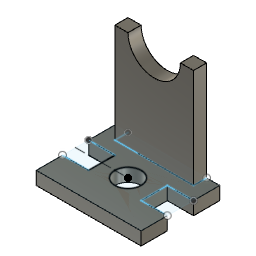
Model 5 (Autodesk Fusion 360 design; units mm, degrees)
Autodesk Fusion 360 part; units mm, degrees
sketch "Sketch15" plane through (0, 0, 0) normal (0, 0, 1) x (1, 0, 0)
  line L0 (0, 0) -> (200, 0)
  line L1 (200, 0) -> (200, 150)
  line L2 (200, 150) -> (0, 150)
  line L3 (0, 150) -> (0, 0)
  dimension "d98" = 200
  dimension "d99" = 150
  constraint horizontal L0
  constraint vertical L1
  constraint horizontal L2
  constraint vertical L3
  constraint coincident L0.start L3.end
  measures "d98" distance of L0.start L0.end
  measures "d99" distance of L0.start L2.end
extrude "Extrude13" add sketch "Sketch15" along normal blind 25
sketch "Sketch16" plane through (0, 0, 25) normal (0, 0, 1) x (-1, 0, 0)
  line L0 (0, -150) -> (0, 0)
  line L1 (0, 0) -> (-200, 0)
  line L2 (-200, 0) -> (-200, -150)
  line L3 (-200, -150) -> (0, -150)
  line L4 (-200, -50) -> (-150, -50)
  line L5 (-150, -50) -> (-150, -100)
  line L6 (-150, -100) -> (-200, -100)
  line L7 (0, -100) -> (-50, -100)
  line L8 (-50, -100) -> (-50, -50)
  line L9 (-50, -50) -> (0, -50)
  line L10 (0, -75) -> (-100, -75) construction
  circle A0 centre (-100, -75) radius 25
  line L11 (-175, -150) -> (-175, -125)
  line L12 (-175, -125) -> (-25, -125)
  line L13 (-25, -125) -> (-25, -150)
  dimension "d103" = 50
  dimension "d104" = 50
  dimension "d105" = 50
  dimension "d106" = 50
  dimension "d107" = 50
  dimension "d108" = 100
  dimension "d109" = 50
  dimension "d111" = 25
  dimension "d112" = 150
  constraint perpendicular L4 L5
  constraint coincident L2 L6.end
  constraint perpendicular L2 L6
  constraint coincident L0 L7.start
  constraint perpendicular L0 L7
  constraint perpendicular L7 L8
  constraint perpendicular L8 L9
  constraint midpoint L0 L10.start
  constraint perpendicular L8 L10
  constraint coincident L10.end A0.centre
  constraint perpendicular L11 L12
  constraint coincident L3 L13.end
  constraint perpendicular L3 L13
  measures "d103" distance of L4.start L4.end
  measures "d104" distance of L4.end L5.end
  measures "d105" distance of L7.start L7.end
  measures "d106" distance of L7.end L8.end
  measures "d107" distance of L8.end L9.end
  measures "d108" distance of L10.start L10.end
  measures "d109" diameter of A0
  measures "d111" distance of L11.start L11.end
  measures "d112" distance of L11.end L12.end
extrude "Extrude14" cut sketch "Sketch16" against normal blind 25 contours L0 L7 L8 L9 | L2 L4 L5 L6
extrude "Extrude15" cut sketch "Sketch16" against normal blind 25 contours A0
extrude "Extrude16" add sketch "Sketch16" along normal blind 190 contours L3 L11 L12 L13
sketch "Sketch17" plane through (0, 125, 0) normal (0, -1, 0) x (1, 0, 0)
  line L0 (25, 25) -> (175, 25)
  line L1 (175, 25) -> (175, 215)
  line L2 (175, 215) -> (25, 215)
  line L3 (25, 215) -> (25, 25)
  line L4 (25, 215) -> (50, 215) construction
  line L5 (175, 215) -> (150, 215) construction
  arc A0 (50, 215) -> (150, 215) centre (100, 215) ccw
  dimension "d119" = 25
  dimension "d120" = 25
  dimension "d121" = 100
  constraint coincident L2.end L3.start
  constraint perpendicular L3 L4
  constraint coincident L1.end L2.start
  constraint perpendicular L1 L5
  constraint midpoint L2 A0.centre
  measures "d119" distance of L2.end L4.end
  measures "d120" distance of L1.end L5.end
  measures "d121" diameter of A0
extrude "Extrude17" cut sketch "Sketch17" against normal blind 25 contours L2 A0
